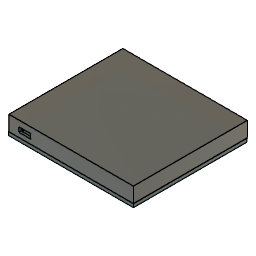
F.R.I.D.A.Y. PAD (Autodesk Fusion 360 design; units mm, degrees)
part number: 2026-08-07-09-18-49-499
Autodesk Fusion 360 part; units mm, degrees
sketch "Sketch1" plane through (0, 0, 0) normal (0, 0, 1) x (1, 0, 0)
  line L0 (-81.4597, 48.1043) -> (25.3403, 48.1043)
  line L1 (25.3403, 48.1043) -> (25.3403, -49.6927)
  line L2 (25.3403, -49.6927) -> (-81.4597, -49.6927)
  line L3 (-81.4597, -49.6927) -> (-81.4597, 48.1043)
  dimension "d1" = 106.8
  constraint horizontal L0
  constraint vertical L1
  constraint horizontal L2
  constraint vertical L3
  measures "d1" distance of L0.start L0.end
extrude "Extrude1" add sketch "Sketch1" along normal blind 13 makes body 1
shell "Shell1" thickness 2 removed faces 1 at (-45.8597, 15.5053, 0) on bodies 1
sketch "Sketch2" plane through (0, 0, 0) normal (0, 0, 1) x (1, 0, 0)
  line L0 (-81.6866, 47.6505) -> (25.4136, 47.6505)
  line L1 (25.4136, 47.6505) -> (25.4136, -49.6927)
  line L2 (25.4136, -49.6927) -> (-81.6866, -49.6927)
  line L3 (-81.6866, -49.6927) -> (-81.6866, 47.6505)
  constraint horizontal L0
  constraint vertical L1
  constraint horizontal L2
  constraint vertical L3
extrude "Extrude2" add sketch "Sketch2" against normal blind 3 separate body makes body 2
sketch "Sketch3" plane through (0, 0, -3) normal (0, 0, -1) x (1, 0, 0)
  line L0 (25.4136, 49.6927) -> (-81.6866, 49.6927)
  line L1 (-81.6866, 49.6927) -> (-81.6866, -47.6505)
  line L2 (-81.6866, -47.6505) -> (25.4136, -47.6505)
  line L3 (25.4136, -47.6505) -> (25.4136, 49.6927)
  line L4 (7.4719, -40.6164) -> (-6.5281, -40.6164)
  line L5 (-6.5281, -40.6164) -> (-6.5281, -26.5481)
  line L6 (-6.5281, -26.5481) -> (7.4719, -26.5481)
  line L7 (7.4719, -26.5481) -> (7.4719, -40.6164)
  line L8 (7.5365, -20.6868) -> (-6.5281, -20.6868)
  line L9 (-6.5281, -20.6868) -> (-6.5281, -6.6868)
  line L10 (-6.5281, -6.6868) -> (7.5365, -6.6868)
  line L11 (7.5365, -6.6868) -> (7.5365, -20.6868)
  line L12 (7.5365, 0.6425) -> (-6.5281, 0.6425)
  line L13 (-6.5281, 0.6425) -> (-6.5281, 14.6425)
  line L14 (-6.5281, 14.6425) -> (7.5365, 14.6425)
  line L15 (7.5365, 14.6425) -> (7.5365, 0.6425)
  line L16 (-21.1185, -40.3895) -> (-35.1185, -40.3895)
  line L17 (-21.0538, 14.8694) -> (-21.0538, 0.8694)
  line L18 (-35.1185, -20.4599) -> (-35.1185, -6.4599)
  line L19 (-21.1185, -26.3212) -> (-21.1185, -40.3895)
  line L20 (-35.1185, 14.8694) -> (-21.0538, 14.8694)
  line L21 (-21.0538, -20.4599) -> (-35.1185, -20.4599)
  line L22 (-21.0538, 0.8694) -> (-35.1185, 0.8694)
  line L23 (-21.0538, -6.4599) -> (-21.0538, -20.4599)
  line L24 (-35.1185, -26.3212) -> (-21.1185, -26.3212)
  line L25 (-35.1185, -6.4599) -> (-21.0538, -6.4599)
  line L26 (-35.1185, 0.8694) -> (-35.1185, 14.8694)
  line L27 (-35.1185, -40.3895) -> (-35.1185, -26.3212)
  line L28 (7.4719, -40.6164) -> (-6.5281, -40.6164)
  line L29 (7.5365, 14.6425) -> (7.5365, 0.6425)
  line L30 (-6.5281, -20.6868) -> (-6.5281, -6.6868)
  line L31 (7.4719, -26.5481) -> (7.4719, -40.6164)
  line L32 (-6.5281, 14.6425) -> (7.5365, 14.6425)
  line L33 (7.5365, -20.6868) -> (-6.5281, -20.6868)
  line L34 (7.5365, 0.6425) -> (-6.5281, 0.6425)
  line L35 (7.5365, -6.6868) -> (7.5365, -20.6868)
  line L36 (-6.5281, -26.5481) -> (7.4719, -26.5481)
  line L37 (-6.5281, -6.6868) -> (7.5365, -6.6868)
  line L38 (-6.5281, 0.6425) -> (-6.5281, 14.6425)
  line L39 (-6.5281, -40.6164) -> (-6.5281, -26.5481)
  line L40 (-49.7088, -40.1626) -> (-63.7088, -40.1626)
  line L41 (-63.7088, -20.233) -> (-63.7088, -6.233)
  line L42 (-49.7088, -26.0943) -> (-49.7088, -40.1626)
  line L43 (-49.6441, -20.233) -> (-63.7088, -20.233)
  line L44 (-49.6441, -6.233) -> (-49.6441, -20.233)
  line L45 (-63.7088, -26.0943) -> (-49.7088, -26.0943)
  line L46 (-63.7088, -6.233) -> (-49.6441, -6.233)
  line L47 (-63.7088, -40.1626) -> (-63.7088, -26.0943)
  dimension "d7" = 14
  dimension "d8" = 14
  dimension "d9" = 14
  dimension "d10" = 14
  dimension "d11" = 14
  dimension "d12" = 14
  dimension "d13" = 14
  dimension "d14" = 14
  dimension "d15" = 14
  dimension "d16" = 14
  dimension "d17" = 14
  constraint horizontal L4
  constraint vertical L5
  constraint horizontal L6
  constraint vertical L7
  constraint horizontal L8
  constraint vertical L9
  constraint horizontal L10
  constraint vertical L11
  constraint horizontal L12
  constraint vertical L13
  constraint horizontal L14
  constraint vertical L15
  constraint horizontal L16
  constraint vertical L27
  constraint horizontal L24
  constraint vertical L19
  constraint horizontal L21
  constraint vertical L18
  constraint horizontal L25
  constraint vertical L23
  constraint horizontal L22
  constraint vertical L26
  constraint horizontal L20
  constraint vertical L17
  constraint horizontal L28
  constraint vertical L39
  constraint horizontal L36
  constraint vertical L31
  constraint horizontal L33
  constraint vertical L30
  constraint horizontal L37
  constraint vertical L35
  constraint horizontal L34
  constraint vertical L38
  constraint horizontal L32
  constraint vertical L29
  constraint horizontal L40
  constraint vertical L47
  constraint horizontal L45
  constraint vertical L42
  constraint horizontal L43
  constraint vertical L41
  constraint horizontal L46
  constraint vertical L44
  measures "d7" distance of L4.start L4.end
  measures "d8" distance of L8.start L10.end
  measures "d9" distance of L12.start L14.end
  measures "d10" distance of L16.end L16.start
  measures "d11" distance of L21.start L23.start
  measures "d12" distance of L17.end L17.start
  measures "d13" distance of L4.end L4.start
  measures "d14" distance of L8.start L10.end
  measures "d15" distance of L12.start L14.end
  measures "d16" distance of L40.end L40.start
  measures "d17" distance of L43.start L44.start
sketch "Sketch4" plane through (0, 0, -3) normal (0, 0, -1) x (1, 0, 0)
  circle A0 centre (-56.3569, 8.6145) radius 4
  dimension "d19" = 8
  measures "d19" diameter of A0
extrude "Extrude3" cut sketch "Sketch3" sketch "Sketch4" against normal blind 5 contours L4 L5 L6 L7 L28 L31 L36 L39 | L8 L9 L10 L11 L30 L33 L35 L37 | L12 L13 L14 L15 L29 L32 L34 L38 | L16 L19 L24 L27 | L17 L20 L22 L26 | L18 L21 L23 L25 | L40 L42 L45 L47 | L41 L43 L44 L46 of sketch 2 bodies 2
sketch "Sketch5" plane through (0, 0, -3) normal (0, 0, -1) x (1, 0, 0)
  line L0 (25.4136, 49.6927) -> (-81.6866, 49.6927)
  line L1 (-81.6866, 49.6927) -> (-81.6866, -47.6505)
  line L2 (-81.6866, -47.6505) -> (25.4136, -47.6505)
  line L3 (25.4136, -47.6505) -> (25.4136, 49.6927)
  circle A0 centre (-56.3569, 8.6145) radius 4
  line L4 (7.5365, -20.6868) -> (-6.5281, -20.6868)
  line L5 (-6.5281, -20.6868) -> (-6.5281, -6.6868)
  line L6 (-6.5281, -6.6868) -> (7.5365, -6.6868)
  line L7 (7.5365, -6.6868) -> (7.5365, -20.6868)
  line L8 (-21.1185, -26.3212) -> (-21.1185, -40.3895)
  line L9 (-21.1185, -40.3895) -> (-35.1185, -40.3895)
  line L10 (-35.1185, -40.3895) -> (-35.1185, -26.3212)
  line L11 (-35.1185, -26.3212) -> (-21.1185, -26.3212)
  line L12 (7.5365, 14.6425) -> (7.5365, 0.6425)
  line L13 (7.5365, 0.6425) -> (-6.5281, 0.6425)
  line L14 (-6.5281, 0.6425) -> (-6.5281, 14.6425)
  line L15 (-6.5281, 14.6425) -> (7.5365, 14.6425)
  line L16 (-49.7088, -26.0943) -> (-49.7088, -40.1626)
  line L17 (-49.7088, -40.1626) -> (-63.7088, -40.1626)
  line L18 (-63.7088, -40.1626) -> (-63.7088, -26.0943)
  line L19 (-63.7088, -26.0943) -> (-49.7088, -26.0943)
  line L20 (-21.0538, 14.8694) -> (-21.0538, 0.8694)
  line L21 (-21.0538, 0.8694) -> (-35.1185, 0.8694)
  line L22 (-35.1185, 0.8694) -> (-35.1185, 14.8694)
  line L23 (-35.1185, 14.8694) -> (-21.0538, 14.8694)
  line L24 (-21.0538, -20.4599) -> (-35.1185, -20.4599)
  line L25 (-35.1185, -20.4599) -> (-35.1185, -6.4599)
  line L26 (-35.1185, -6.4599) -> (-21.0538, -6.4599)
  line L27 (-21.0538, -6.4599) -> (-21.0538, -20.4599)
  line L28 (7.4719, -26.5481) -> (7.4719, -40.6164)
  line L29 (7.4719, -40.6164) -> (-6.5281, -40.6164)
  line L30 (-6.5281, -40.6164) -> (-6.5281, -26.5481)
  line L31 (-6.5281, -26.5481) -> (7.4719, -26.5481)
  line L32 (-49.6441, -20.233) -> (-63.7088, -20.233)
  line L33 (-63.7088, -20.233) -> (-63.7088, -6.233)
  line L34 (-63.7088, -6.233) -> (-49.6441, -6.233)
  line L35 (-49.6441, -6.233) -> (-49.6441, -20.233)
  line L36 (-0.243, 27.4558) -> (-26.1104, 27.4558)
  line L37 (-26.1104, 27.4558) -> (-26.1104, 40.4558)
  line L38 (-26.1104, 40.4558) -> (-0.243, 40.4558)
  line L39 (-0.243, 40.4558) -> (-0.243, 27.4558)
  dimension "d22" = 13
  constraint horizontal L36
  constraint vertical L37
  constraint horizontal L38
  constraint vertical L39
  measures "d22" distance of L36.start L38.end
extrude "Extrude4" cut sketch "Sketch5" against normal blind 5 contours L36 L37 L38 L39 bodies 2
sketch "Sketch6" plane through (0, 0, -3) normal (0, 0, -1) x (1, 0, 0)
  line L0 (-49.6441, -20.233) -> (-63.7088, -20.233)
  line L1 (-63.7088, -20.233) -> (-63.7088, -6.233)
  line L2 (-63.7088, -6.233) -> (-49.6441, -6.233)
  line L3 (-49.6441, -6.233) -> (-49.6441, -20.233)
  line L4 (7.4719, -26.5481) -> (7.4719, -40.6164)
  line L5 (7.4719, -40.6164) -> (-6.5281, -40.6164)
  line L6 (-6.5281, -40.6164) -> (-6.5281, -26.5481)
  line L7 (-6.5281, -26.5481) -> (7.4719, -26.5481)
  line L8 (-21.0538, -20.4599) -> (-35.1185, -20.4599)
  line L9 (-35.1185, -20.4599) -> (-35.1185, -6.4599)
  line L10 (-35.1185, -6.4599) -> (-21.0538, -6.4599)
  line L11 (-21.0538, -6.4599) -> (-21.0538, -20.4599)
  line L12 (-21.0538, 14.8694) -> (-21.0538, 0.8694)
  line L13 (-21.0538, 0.8694) -> (-35.1185, 0.8694)
  line L14 (-35.1185, 0.8694) -> (-35.1185, 14.8694)
  line L15 (-35.1185, 14.8694) -> (-21.0538, 14.8694)
  line L16 (-49.7088, -26.0943) -> (-49.7088, -40.1626)
  line L17 (-49.7088, -40.1626) -> (-63.7088, -40.1626)
  line L18 (-63.7088, -40.1626) -> (-63.7088, -26.0943)
  line L19 (-63.7088, -26.0943) -> (-49.7088, -26.0943)
  line L20 (7.5365, 14.6425) -> (7.5365, 0.6425)
  line L21 (7.5365, 0.6425) -> (-6.5281, 0.6425)
  line L22 (-6.5281, 0.6425) -> (-6.5281, 14.6425)
  line L23 (-6.5281, 14.6425) -> (7.5365, 14.6425)
  line L24 (-21.1185, -26.3212) -> (-21.1185, -40.3895)
  line L25 (-21.1185, -40.3895) -> (-35.1185, -40.3895)
  line L26 (-35.1185, -40.3895) -> (-35.1185, -26.3212)
  line L27 (-35.1185, -26.3212) -> (-21.1185, -26.3212)
  line L28 (7.5365, -20.6868) -> (-6.5281, -20.6868)
  line L29 (-6.5281, -20.6868) -> (-6.5281, -6.6868)
  line L30 (-6.5281, -6.6868) -> (7.5365, -6.6868)
  line L31 (7.5365, -6.6868) -> (7.5365, -20.6868)
  circle A0 centre (-56.3569, 8.6145) radius 4
  line L32 (25.4136, 49.6927) -> (-81.6866, 49.6927)
  line L33 (-81.6866, 49.6927) -> (-81.6866, -47.6505)
  line L34 (-81.6866, -47.6505) -> (25.4136, -47.6505)
  line L35 (25.4136, -47.6505) -> (25.4136, 49.6927)
  line L36 (-26.1104, 27.4558) -> (-26.1104, 40.4558)
  line L37 (-26.1104, 40.4558) -> (-0.243, 40.4558)
  line L38 (-0.243, 40.4558) -> (-0.243, 27.4558)
  line L39 (-0.243, 27.4558) -> (-26.1104, 27.4558)
sketch "Sketch7" plane through (0, 0, -3) normal (0, 0, -1) x (1, 0, 0)
sketch "Sketch8" plane through (0, 0, -3) normal (0, 0, -1) x (1, 0, 0)
sketch "Sketch9" plane through (0, -49.6927, 0) normal (0, -1, 0) x (1, 0, 0)
  line L0 (-81.4597, 0) -> (25.3403, 0)
  line L1 (25.3403, 0) -> (25.3403, 13)
  line L2 (25.3403, 13) -> (-81.4597, 13)
  line L3 (-81.4597, 13) -> (-81.4597, 0)
  line L4 (-62.6425, 7.9418) -> (-72.8533, 7.9418)
  line L5 (-72.8533, 7.9418) -> (-72.8533, 3.9418)
  line L6 (-72.8533, 3.9418) -> (-62.6425, 3.9418)
  line L7 (-62.6425, 3.9418) -> (-62.6425, 7.9418)
  dimension "d26" = 4
  constraint horizontal L4
  constraint vertical L5
  constraint horizontal L6
  constraint vertical L7
  measures "d26" distance of L4.start L6.end
extrude "Extrude5" cut sketch "Sketch9" against normal blind 5 contours L4 L5 L6 L7 bodies 1
sketch "Sketch10" plane through (0, 0, -3) normal (0, 0, -1) x (1, 0, 0)
  circle A0 centre (-76.6946, -42.8855) radius 1.6
  circle A1 centre (-76.6946, 44.1487) radius 1.6
  circle A2 centre (20.5825, -42.8855) radius 1.6
  circle A3 centre (20.8094, 43.6948) radius 1.6
  dimension "d29" = 3.2
  dimension "d30" = 3.2
  dimension "d31" = 3.2
  dimension "d32" = 3.2
  measures "d29" diameter of A0
  measures "d30" diameter of A1
  measures "d31" diameter of A2
  measures "d32" diameter of A3
extrude "Extrude6" cut sketch "Sketch10" against normal blind 15 contours A3 bodies 1 2
sketch "Sketch11" plane through (0, 0, -3) normal (0, 0, -1) x (1, 0, 0)
  circle A0 centre (-76.9216, -43.2571) radius 1.6
  point P0 (-76.9216, -43.2571)
  point P1 (-76.9216, 44.9276)
  point P2 (21.2632, -43.0302)
  dimension "d35" = 3.2
  measures "d35" diameter of A0
extrude "Extrude7" cut sketch "Sketch11" against normal blind 15 bodies 1 2
sketch "Sketch12" plane through (0, 0, -3) normal (0, 0, -1) x (1, 0, 0)
  circle A0 centre (21.1024, -43.3393) radius 1.6
  dimension "d38" = 3.2
  measures "d38" diameter of A0
extrude "Extrude8" cut sketch "Sketch12" against normal blind 15 bodies 1 2
sketch "Sketch13" plane through (0, 0, -3) normal (0, 0, -1) x (1, 0, 0)
  circle A0 centre (-76.4677, 44.2469) radius 1.6
  dimension "d41" = 3.2
  measures "d41" diameter of A0
extrude "Extrude9" cut sketch "Sketch13" against normal blind 15 bodies 1 2
